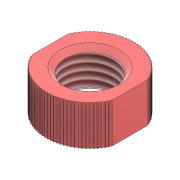
# Autodesk Inventor part: Tuerca_interruptor_BlueRobotics
Saved by Autodesk Inventor 2022.3 (Build 263350000, 350)
## iProperties
Created: 2023-07-17
Part Number: Tuerca_interruptor_BlueRobotics
Material: Genérico
Document SubType Name: Modeling
Designer: Usuario
Density: 1 g/cm^3
Appearance: Valor por defecto
Author: Usuario
Autodesk Inventor part; units mm, degrees
ref_plane "YZ Plane" through (0, 0, 0) normal (1, 0, 0) x (0, 1, 0)
ref_plane "XZ Plane" through (0, 0, 0) normal (0, 1, 0) x (-1, 0, 0)
ref_plane "XY Plane" through (0, 0, 0) normal (0, 0, 1) x (1, 0, 0)
sketch "Boceto1" plane through (0, 0, 0) normal (0, 1, 0) x (-1, 0, 0)
  line L0 (8, -3.5618) -> (8, 3.5618)
  arc A0 (7.8902, 3.9678) -> (8, 3.5618) centre (8.0756, 3.8001) ccw
  arc A1 (7.8902, 3.9678) -> (7.8478, 4.0511) centre (7.8531, 4.0014) ccw
  arc A2 (7.6255, 4.4554) -> (7.8478, 4.0511) centre (7.821, 4.2997) ccw
  arc A3 (7.6255, 4.4554) -> (7.5779, 4.5359) centre (7.5864, 4.4866) ccw
  arc A4 (7.3307, 4.9254) -> (7.5779, 4.5359) centre (7.5356, 4.7823) ccw
  arc A5 (7.3307, 4.9254) -> (7.2782, 5.0027) centre (7.2897, 4.9541) ccw
  arc A6 (7.007, 5.376) -> (7.2782, 5.0027) centre (7.2205, 5.246) ccw
  arc A7 (7.007, 5.376) -> (6.9497, 5.4499) centre (6.9643, 5.402) ccw
  arc A8 (6.6556, 5.8054) -> (6.9497, 5.4499) centre (6.8768, 5.689) ccw
  arc A9 (6.6556, 5.8054) -> (6.5938, 5.8755) centre (6.6113, 5.8287) ccw
  arc A10 (6.2779, 6.2118) -> (6.5938, 5.8755) centre (6.506, 6.1096) ccw
  arc A11 (6.2779, 6.2118) -> (6.2118, 6.2779) centre (6.2323, 6.2323) ccw
  arc A12 (5.8755, 6.5938) -> (6.2118, 6.2779) centre (6.1096, 6.506) ccw
  arc A13 (5.8755, 6.5938) -> (5.8054, 6.6556) centre (5.8287, 6.6113) ccw
  arc A14 (5.4499, 6.9497) -> (5.8054, 6.6556) centre (5.689, 6.8768) ccw
  arc A15 (5.4499, 6.9497) -> (5.376, 7.007) centre (5.402, 6.9643) ccw
  arc A16 (5.0027, 7.2782) -> (5.376, 7.007) centre (5.246, 7.2205) ccw
  arc A17 (5.0027, 7.2782) -> (4.9254, 7.3307) centre (4.9541, 7.2897) ccw
  arc A18 (4.5359, 7.5779) -> (4.9254, 7.3307) centre (4.7823, 7.5356) ccw
  arc A19 (4.5359, 7.5779) -> (4.4554, 7.6255) centre (4.4866, 7.5864) ccw
  arc A20 (4.0511, 7.8478) -> (4.4554, 7.6255) centre (4.2997, 7.821) ccw
  arc A21 (4.0511, 7.8478) -> (3.9678, 7.8902) centre (4.0014, 7.8531) ccw
  arc A22 (3.5503, 8.0867) -> (3.9678, 7.8902) centre (3.8001, 8.0756) ccw
  arc A23 (3.5503, 8.0867) -> (3.4646, 8.1238) centre (3.5004, 8.0889) ccw
  arc A24 (3.0356, 8.2936) -> (3.4646, 8.1238) centre (3.2855, 8.2983) ccw
  arc A25 (3.0356, 8.2936) -> (2.9476, 8.3253) centre (2.9856, 8.2927) ccw
  arc A26 (2.5088, 8.4679) -> (2.9476, 8.3253) centre (2.758, 8.4882) ccw
  arc A27 (2.5088, 8.4679) -> (2.4191, 8.494) centre (2.459, 8.4638) ccw
  arc A28 (1.9721, 8.6087) -> (2.4191, 8.494) centre (2.2196, 8.6446) ccw
  arc A29 (1.9721, 8.6087) -> (1.881, 8.6291) centre (1.9227, 8.6015) ccw
  arc A30 (1.4277, 8.7155) -> (1.881, 8.6291) centre (1.6724, 8.7669) ccw
  arc A31 (1.4277, 8.7155) -> (1.3354, 8.7302) centre (1.3788, 8.7053) ccw
  arc A32 (0.8776, 8.788) -> (1.3354, 8.7302) centre (1.1186, 8.8546) ccw
  arc A33 (0.8776, 8.788) -> (0.7846, 8.7968) centre (0.8295, 8.7747) ccw
  arc A34 (0.3241, 8.8258) -> (0.7846, 8.7968) centre (0.5604, 8.9074) ccw
  arc A35 (0.3241, 8.8258) -> (0.2307, 8.8287) centre (0.2768, 8.8094) ccw
  arc A36 (-0.2307, 8.8287) -> (0.2307, 8.8287) centre (0, 8.925) ccw
  arc A37 (-0.2307, 8.8287) -> (-0.3241, 8.8258) centre (-0.2768, 8.8094) ccw
  arc A38 (-0.7846, 8.7968) -> (-0.3241, 8.8258) centre (-0.5604, 8.9074) ccw
  arc A39 (-0.7846, 8.7968) -> (-0.8776, 8.788) centre (-0.8295, 8.7747) ccw
  arc A40 (-1.3354, 8.7302) -> (-0.8776, 8.788) centre (-1.1186, 8.8546) ccw
  arc A41 (-1.3354, 8.7302) -> (-1.4277, 8.7155) centre (-1.3788, 8.7053) ccw
  arc A42 (-1.881, 8.6291) -> (-1.4277, 8.7155) centre (-1.6724, 8.7669) ccw
  arc A43 (-1.881, 8.6291) -> (-1.9721, 8.6087) centre (-1.9227, 8.6015) ccw
  arc A44 (-2.4191, 8.494) -> (-1.9721, 8.6087) centre (-2.2196, 8.6446) ccw
  arc A45 (-2.4191, 8.494) -> (-2.5088, 8.4679) centre (-2.459, 8.4638) ccw
  arc A46 (-2.9476, 8.3253) -> (-2.5088, 8.4679) centre (-2.758, 8.4882) ccw
  arc A47 (-2.9476, 8.3253) -> (-3.0356, 8.2936) centre (-2.9856, 8.2927) ccw
  arc A48 (-3.4646, 8.1238) -> (-3.0356, 8.2936) centre (-3.2855, 8.2983) ccw
  arc A49 (-3.4646, 8.1238) -> (-3.5503, 8.0867) centre (-3.5004, 8.0889) ccw
  arc A50 (-3.9678, 7.8902) -> (-3.5503, 8.0867) centre (-3.8001, 8.0756) ccw
  arc A51 (-3.9678, 7.8902) -> (-4.0511, 7.8478) centre (-4.0014, 7.8531) ccw
  arc A52 (-4.4554, 7.6255) -> (-4.0511, 7.8478) centre (-4.2997, 7.821) ccw
  arc A53 (-4.4554, 7.6255) -> (-4.5359, 7.5779) centre (-4.4866, 7.5864) ccw
  arc A54 (-4.9254, 7.3307) -> (-4.5359, 7.5779) centre (-4.7823, 7.5356) ccw
  arc A55 (-4.9254, 7.3307) -> (-5.0027, 7.2782) centre (-4.9541, 7.2897) ccw
  arc A56 (-5.376, 7.007) -> (-5.0027, 7.2782) centre (-5.246, 7.2205) ccw
  arc A57 (-5.376, 7.007) -> (-5.4499, 6.9497) centre (-5.402, 6.9643) ccw
  arc A58 (-5.8054, 6.6556) -> (-5.4499, 6.9497) centre (-5.689, 6.8768) ccw
  arc A59 (-5.8054, 6.6556) -> (-5.8755, 6.5938) centre (-5.8287, 6.6113) ccw
  arc A60 (-6.2118, 6.2779) -> (-5.8755, 6.5938) centre (-6.1096, 6.506) ccw
  arc A61 (-6.2118, 6.2779) -> (-6.2779, 6.2118) centre (-6.2323, 6.2323) ccw
  arc A62 (-6.5938, 5.8755) -> (-6.2779, 6.2118) centre (-6.506, 6.1096) ccw
  arc A63 (-6.5938, 5.8755) -> (-6.6556, 5.8054) centre (-6.6113, 5.8287) ccw
  arc A64 (-6.9497, 5.4499) -> (-6.6556, 5.8054) centre (-6.8768, 5.689) ccw
  arc A65 (-6.9497, 5.4499) -> (-7.007, 5.376) centre (-6.9643, 5.402) ccw
  arc A66 (-7.2782, 5.0027) -> (-7.007, 5.376) centre (-7.2205, 5.246) ccw
  arc A67 (-7.2782, 5.0027) -> (-7.3307, 4.9254) centre (-7.2897, 4.9541) ccw
  arc A68 (-7.5779, 4.5359) -> (-7.3307, 4.9254) centre (-7.5356, 4.7823) ccw
  arc A69 (-7.5779, 4.5359) -> (-7.6255, 4.4554) centre (-7.5864, 4.4866) ccw
  arc A70 (-7.8478, 4.0511) -> (-7.6255, 4.4554) centre (-7.821, 4.2997) ccw
  arc A71 (-7.8478, 4.0511) -> (-7.8902, 3.9678) centre (-7.8531, 4.0014) ccw
  arc A72 (-8, 3.5618) -> (-7.8902, 3.9678) centre (-8.0756, 3.8001) ccw
  line L1 (-8, 3.5618) -> (-8, -3.5618)
  arc A73 (-7.8902, -3.9678) -> (-8, -3.5618) centre (-8.0756, -3.8001) ccw
  arc A74 (-7.8902, -3.9678) -> (-7.8478, -4.0511) centre (-7.8531, -4.0014) ccw
  arc A75 (-7.6255, -4.4554) -> (-7.8478, -4.0511) centre (-7.821, -4.2997) ccw
  arc A76 (-7.6255, -4.4554) -> (-7.5779, -4.5359) centre (-7.5864, -4.4866) ccw
  arc A77 (-7.3307, -4.9254) -> (-7.5779, -4.5359) centre (-7.5356, -4.7823) ccw
  arc A78 (-7.3307, -4.9254) -> (-7.2782, -5.0027) centre (-7.2897, -4.9541) ccw
  arc A79 (-7.007, -5.376) -> (-7.2782, -5.0027) centre (-7.2205, -5.246) ccw
  arc A80 (-7.007, -5.376) -> (-6.9497, -5.4499) centre (-6.9643, -5.402) ccw
  arc A81 (-6.6556, -5.8054) -> (-6.9497, -5.4499) centre (-6.8768, -5.689) ccw
  arc A82 (-6.6556, -5.8054) -> (-6.5938, -5.8755) centre (-6.6113, -5.8287) ccw
  arc A83 (-6.2779, -6.2118) -> (-6.5938, -5.8755) centre (-6.506, -6.1096) ccw
  arc A84 (-6.2779, -6.2118) -> (-6.2118, -6.2779) centre (-6.2323, -6.2323) ccw
  arc A85 (-5.8755, -6.5938) -> (-6.2118, -6.2779) centre (-6.1096, -6.506) ccw
  arc A86 (-5.8755, -6.5938) -> (-5.8054, -6.6556) centre (-5.8287, -6.6113) ccw
  arc A87 (-5.4499, -6.9497) -> (-5.8054, -6.6556) centre (-5.689, -6.8768) ccw
  arc A88 (-5.4499, -6.9497) -> (-5.376, -7.007) centre (-5.402, -6.9643) ccw
  arc A89 (-5.0027, -7.2782) -> (-5.376, -7.007) centre (-5.246, -7.2205) ccw
  arc A90 (-5.0027, -7.2782) -> (-4.9254, -7.3307) centre (-4.9541, -7.2897) ccw
  arc A91 (-4.5359, -7.5779) -> (-4.9254, -7.3307) centre (-4.7823, -7.5356) ccw
  arc A92 (-4.5359, -7.5779) -> (-4.4554, -7.6255) centre (-4.4866, -7.5864) ccw
  arc A93 (-4.0511, -7.8478) -> (-4.4554, -7.6255) centre (-4.2997, -7.821) ccw
  arc A94 (-4.0511, -7.8478) -> (-3.9678, -7.8902) centre (-4.0014, -7.8531) ccw
  arc A95 (-3.5503, -8.0867) -> (-3.9678, -7.8902) centre (-3.8001, -8.0756) ccw
  arc A96 (-3.5503, -8.0867) -> (-3.4646, -8.1238) centre (-3.5004, -8.0889) ccw
  arc A97 (-3.0356, -8.2936) -> (-3.4646, -8.1238) centre (-3.2855, -8.2983) ccw
  arc A98 (-3.0356, -8.2936) -> (-2.9476, -8.3253) centre (-2.9856, -8.2927) ccw
  arc A99 (-2.5088, -8.4679) -> (-2.9476, -8.3253) centre (-2.758, -8.4882) ccw
  arc A100 (-2.5088, -8.4679) -> (-2.4191, -8.494) centre (-2.459, -8.4638) ccw
  arc A101 (-1.9721, -8.6087) -> (-2.4191, -8.494) centre (-2.2196, -8.6446) ccw
  arc A102 (-1.9721, -8.6087) -> (-1.881, -8.6291) centre (-1.9227, -8.6015) ccw
  arc A103 (-1.4277, -8.7155) -> (-1.881, -8.6291) centre (-1.6724, -8.7669) ccw
  arc A104 (-1.4277, -8.7155) -> (-1.3354, -8.7302) centre (-1.3788, -8.7053) ccw
  arc A105 (-0.8776, -8.788) -> (-1.3354, -8.7302) centre (-1.1186, -8.8546) ccw
  arc A106 (-0.8776, -8.788) -> (-0.7846, -8.7968) centre (-0.8295, -8.7747) ccw
  arc A107 (-0.3241, -8.8258) -> (-0.7846, -8.7968) centre (-0.5604, -8.9074) ccw
  arc A108 (-0.3241, -8.8258) -> (-0.2307, -8.8287) centre (-0.2768, -8.8094) ccw
  arc A109 (0.2307, -8.8287) -> (-0.2307, -8.8287) centre (0, -8.925) ccw
  arc A110 (0.2307, -8.8287) -> (0.3241, -8.8258) centre (0.2768, -8.8094) ccw
  arc A111 (0.7846, -8.7968) -> (0.3241, -8.8258) centre (0.5604, -8.9074) ccw
  arc A112 (0.7846, -8.7968) -> (0.8776, -8.788) centre (0.8295, -8.7747) ccw
  arc A113 (1.3354, -8.7302) -> (0.8776, -8.788) centre (1.1186, -8.8546) ccw
  arc A114 (1.3354, -8.7302) -> (1.4277, -8.7155) centre (1.3788, -8.7053) ccw
  arc A115 (1.881, -8.6291) -> (1.4277, -8.7155) centre (1.6724, -8.7669) ccw
  arc A116 (1.881, -8.6291) -> (1.9721, -8.6087) centre (1.9227, -8.6015) ccw
  arc A117 (2.4191, -8.494) -> (1.9721, -8.6087) centre (2.2196, -8.6446) ccw
  arc A118 (2.4191, -8.494) -> (2.5088, -8.4679) centre (2.459, -8.4638) ccw
  arc A119 (2.9476, -8.3253) -> (2.5088, -8.4679) centre (2.758, -8.4882) ccw
  arc A120 (2.9476, -8.3253) -> (3.0356, -8.2936) centre (2.9856, -8.2927) ccw
  arc A121 (3.4646, -8.1238) -> (3.0356, -8.2936) centre (3.2855, -8.2983) ccw
  arc A122 (3.4646, -8.1238) -> (3.5503, -8.0867) centre (3.5004, -8.0889) ccw
  arc A123 (3.9678, -7.8902) -> (3.5503, -8.0867) centre (3.8001, -8.0756) ccw
  arc A124 (3.9678, -7.8902) -> (4.0511, -7.8478) centre (4.0014, -7.8531) ccw
  arc A125 (4.4554, -7.6255) -> (4.0511, -7.8478) centre (4.2997, -7.821) ccw
  arc A126 (4.4554, -7.6255) -> (4.5359, -7.5779) centre (4.4866, -7.5864) ccw
  arc A127 (4.9254, -7.3307) -> (4.5359, -7.5779) centre (4.7823, -7.5356) ccw
  arc A128 (4.9254, -7.3307) -> (5.0027, -7.2782) centre (4.9541, -7.2897) ccw
  arc A129 (5.376, -7.007) -> (5.0027, -7.2782) centre (5.246, -7.2205) ccw
  arc A130 (5.376, -7.007) -> (5.4499, -6.9497) centre (5.402, -6.9643) ccw
  arc A131 (5.8054, -6.6556) -> (5.4499, -6.9497) centre (5.689, -6.8768) ccw
  arc A132 (5.8054, -6.6556) -> (5.8755, -6.5938) centre (5.8287, -6.6113) ccw
  arc A133 (6.2118, -6.2779) -> (5.8755, -6.5938) centre (6.1096, -6.506) ccw
  arc A134 (6.2118, -6.2779) -> (6.2779, -6.2118) centre (6.2323, -6.2323) ccw
  arc A135 (6.5938, -5.8755) -> (6.2779, -6.2118) centre (6.506, -6.1096) ccw
  arc A136 (6.5938, -5.8755) -> (6.6556, -5.8054) centre (6.6113, -5.8287) ccw
  arc A137 (6.9497, -5.4499) -> (6.6556, -5.8054) centre (6.8768, -5.689) ccw
  arc A138 (6.9497, -5.4499) -> (7.007, -5.376) centre (6.9643, -5.402) ccw
  arc A139 (7.2782, -5.0027) -> (7.007, -5.376) centre (7.2205, -5.246) ccw
  arc A140 (7.2782, -5.0027) -> (7.3307, -4.9254) centre (7.2897, -4.9541) ccw
  arc A141 (7.5779, -4.5359) -> (7.3307, -4.9254) centre (7.5356, -4.7823) ccw
  arc A142 (7.5779, -4.5359) -> (7.6255, -4.4554) centre (7.5864, -4.4866) ccw
  arc A143 (7.8478, -4.0511) -> (7.6255, -4.4554) centre (7.821, -4.2997) ccw
  arc A144 (7.8478, -4.0511) -> (7.8902, -3.9678) centre (7.8531, -4.0014) ccw
  arc A145 (8, -3.5618) -> (7.8902, -3.9678) centre (8.0756, -3.8001) ccw
  circle A146 centre (0, 0) radius 5
  dimension "d0" = 10
  constraints: 292 point on circle, 147 centre point, 4 end point, 1 coincident
  measures "d0" diameter of A146
extrude "Extrusión1" add sketch "Boceto1" along normal blind 8
chamfer "Chaflán1" distance 1 angle 45 2 edges at (5, 8, 0) (5, 0, 0)
thread "Rosca1" size "M10x1.5" class "6H" standard "ANSI Metric M Profile" length 6.2
